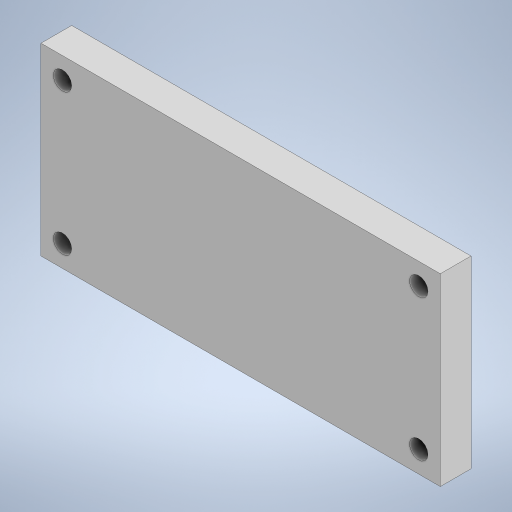
# Autodesk Inventor part: OrangePi
Saved by Autodesk Inventor 2024 (Build 280153000, 153)
## iProperties
Created: 2024-03-12
Part Number: OrangePi
Material: Générique
Document SubType Name: Modeling
Designer: phaly
Density: 1 g/cm^3
Appearance: Par défaut
Author: phaly
Autodesk Inventor part; units mm, degrees
ref_plane "YZ Plane" through (0, 0, 0) normal (1, 0, 0) x (0, 1, 0)
ref_plane "XZ Plane" through (0, 0, 0) normal (0, 1, 0) x (-1, 0, 0)
ref_plane "XY Plane" through (0, 0, 0) normal (0, 0, 1) x (1, 0, 0)
sketch "Esquisse1" plane through (0, 0, 0) normal (0, 0, 1) x (1, 0, 0)
  line L0 (0, 30) -> (65, 30)
  line L1 (65, 30) -> (65, 0)
  line L2 (65, 0) -> (0, 0)
  line L3 (0, 0) -> (0, 30)
  line L4 (-13, 0) -> (78, 0) projected
  line L5 (0, -6) -> (0, 36) projected
  point P0 (0, 0)
  dimension "d0" = 65
  dimension "d1" = 30
  constraints: 8 end point, 2 collinear, 2 parallel, 1 horizontal, 1 perpendicular
  measures "d0" distance of L0.start L0.end
  measures "d1" distance between parallel lines of L2 L0
extrude "Extrusion1" add sketch "Esquisse1" along normal mid plane 5
sketch "Esquisse2" plane through (0, 0, 2.5) normal (0, 0, 1) x (1, 0, 0)
  line L0 (0, 30) -> (0, 0) projected
  line L1 (0, 0) -> (65, 0) projected
  line L2 (65, 30) -> (0, 30) projected
  point P0 (3.5, 26.5)
  point P1 (61.5, 26.5)
  point P2 (61.5, 3.5)
  point P3 (3.5, 3.5)
  dimension "d4" = 58
  dimension "d5" = 23
  dimension "d6" = 23
  dimension "d7" = 58
  dimension "d8" = 3.5
  dimension "d9" = 3.5
  dimension "d10" = 3.5
  dimension "d11" = 3.5
  measures "d4" distance of point (61.5, 26.5) point (3.5, 26.5)
  measures "d5" distance of point (3.5, 3.5) point (3.5, 26.5)
  measures "d6" distance of point (61.5, 3.5) point (61.5, 26.5)
  measures "d7" distance of point (3.5, 3.5) point (61.5, 3.5)
  measures "d8" distance from line of L0 point (3.5, 26.5)
  measures "d9" distance from line of L0 point (3.5, 3.5)
  measures "d10" distance from line of L1 point (3.5, 3.5)
  measures "d11" distance from line of L2 point (61.5, 26.5)
hole "Perçage1" at (3.5, 26.5, 2.5) at (61.5, 26.5, 2.5) at (61.5, 3.5, 2.5) at (3.5, 3.5, 2.5) direction (0, 0, -1) diameter 3 end through all
equation "\"d6\" = d5"
equation "\"d7\" = d4"
equation "\"d9\" = d8"
equation "\"d10\" = d9"
equation "\"d11\" = d8"
